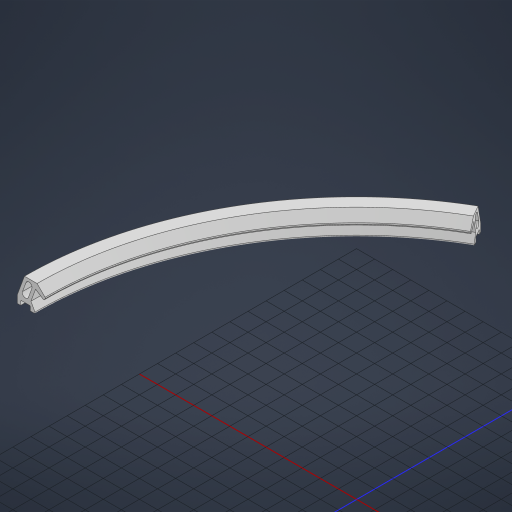
# Autodesk Inventor part: LED-Ring_Element
Saved by Autodesk Inventor 2023.2 (Build 272271030, 271C)
## iProperties
Created: 2023-02-18
Part Number: LED-Ring_Element
Material: Generisch
Document SubType Name: Modeling
Designer: Stefan
Mass: 133.438 g
Surface Area: 652.824 cm^2
Volume: 133.438 cm^3
Density: 1 g/cm^3
Appearance: Vorgabe
Author: Stefan
Autodesk Inventor part; units mm, degrees
ref_plane "YZ Plane" through (0, 0, 0) normal (1, 0, 0) x (0, 1, 0)
ref_plane "XZ Plane" through (0, 0, 0) normal (0, 1, 0) x (-1, 0, 0)
ref_plane "XY Plane" through (0, 0, 0) normal (0, 0, 1) x (1, 0, 0)
sketch "Skizze1" plane through (0, 0, 0) normal (0, 0, 1) x (1, 0, 0)
  arc A0 (-370.4, 125) -> (-371.4, 124) centre (-370.4, 124) ccw
  line L0 (-361.6643, 125) -> (-370.4, 125)
  arc A1 (-360.6643, 124) -> (-361.6643, 125) centre (-361.6643, 124) ccw
  line L1 (-360.6643, 120) -> (-360.6643, 124)
  arc A2 (-346.4361, 138.3117) -> (-345.027, 138.6477) centre (-345.8915, 139.1504) ccw
  line L2 (-344.2357, 140.0086) -> (-345.027, 138.6477)
  arc A3 (-344.2357, 140.0086) -> (-344.3931, 141.2184) centre (-345.1002, 140.5113) ccw
  line L3 (-353.1746, 150) -> (-344.3931, 141.2184)
  line L4 (-367.1746, 150) -> (-353.1746, 150)
  line L5 (-375, 128.5) -> (-367.1746, 150)
  line L6 (-375, 120) -> (-375, 128.5)
  line L7 (-371.4, 120) -> (-375, 120)
  line L8 (-371.4, 124) -> (-371.4, 120)
  line L9 (-357.3008, 147) -> (-364.6666, 147) construction
  line L10 (-364.6666, 147) -> (-371.4, 128.5) construction
  line L11 (0, 0) -> (-360, 0) construction
  line L12 (-356.9218, 138.1504) -> (-345, 0) construction
  line L13 (-356.9218, 138.1504) -> (0, 138.1504) construction
  line L14 (0, 138.1504) -> (0, 0) construction
  line L15 (-360, 129.6932) -> (-360, 0) construction
  line L16 (0, 0) -> (-225, 0) construction
  line L17 (-225, 0) -> (-225, 50) construction
  line L18 (-225, 50) -> (0, 50) construction
  line L19 (0, 50) -> (0, 0) construction
  line L20 (-346.4361, 138.3117) -> (-354.8697, 143.7886)
  line L21 (-360, 129.6932) -> (-355.5655, 121.4749)
  arc A4 (-356.4455, 120) -> (-355.5655, 121.4749) centre (-356.4455, 121) ccw
  line L22 (-225, 0) -> (-345, 0) construction
  line L23 (-345, 0) -> (-345, 35) construction
  line L24 (-345, 35) -> (-225, 35) construction
  line L25 (-225, 35) -> (-225, 0) construction
  line L26 (-356.4455, 120) -> (-360.6643, 120)
  line L27 (-354.8697, 143.7886) -> (-360, 129.6932)
  line L28 (-356.9218, 138.1504) -> (0, 8.2415) construction
  line L29 (-363.6, 129.6932) -> (-357.3008, 147) construction
  line L30 (-360, 129.6932) -> (-374.5657, 129.6932) construction
  line L31 (-363.6, 129.6932) -> (-358.3696, 120) construction
  line L32 (-344.2357, 140.0086) -> (-355.581, 120.4973) construction
  arc A5 (-358.9913, 142.3556) -> (-365.4954, 144.7229) centre (-362.2433, 143.5392) ccw
  arc A6 (-369.2753, 134.3376) -> (-362.7712, 131.9703) centre (-366.0232, 133.1539) ccw
  line L33 (-365.4954, 144.7229) -> (-369.2753, 134.3376)
  line L34 (-358.9913, 142.3556) -> (-362.7712, 131.9703)
  line L35 (-371.4, 120) -> (-371.4, 128.5) construction
  dimension "d1" = 30
  dimension "d5" = 1
  dimension "d6" = 1
  dimension "d9" = 135
  dimension "d14" = 8.5
  dimension "d18" = 360
  dimension "d25" = 50
  dimension "d26" = 225
  dimension "d31" = 14
  dimension "d40" = 3.5
  dimension "d41" = 120
  dimension "d42" = 35
  dimension "d43" = 1
  dimension "d47" = 6
  dimension "d50" = 65.068
  dimension "d54" = 15
  dimension "d55" = 3
  dimension "d59" = 12
  dimension "d60" = 160
  dimension "d61" = 120
  dimension "d63" = 3.6
  dimension "d64" = 3.6
  dimension "d65" = 5
  dimension "d66" = 15
  constraints: 72 end point, 19 tangent, 15 point on circle, 12 point on line, 8 parallel, 7 centre point, 6 horizontal, 5 vertical, 3 perpendicular, 2 collinear, 2 equal radius, 1 horizontal alignment, 4 other
  measures "d1" distance between parallel lines of L7 L4
  measures "d5" radius of A3
  measures "d6" radius of A0
  measures "d9" angle of L3 L4
  measures "d14" distance of L6.start L5.start
  measures "d18" distance of L11.end L11.start
  measures "d25" distance of L16.end L17.end
  measures "d26" distance of L17.end L18.end
  measures "d31" distance of L4.start L3.start
  measures "d40" distance from line of L20.start L3
  measures "d41" distance of L23.end L24.end
  measures "d42" distance of L22.end L23.end
  measures "d43" radius of A4
  measures "d47" distance of L20.end L13.start
  measures "d54" distance of L15.start L20.end
  measures "d55" distance between parallel lines of L4 L9
  measures "d59" angle of L3 L20
  measures "d60" angle of L15 L27
  measures "d61" distance between parallel lines of L11 L26
  measures "d63" distance of L15.start L29.start
  measures "d64" distance between parallel lines of L8 L6
  measures "d65" distance between parallel lines of L0 L7
  measures "d66" distance between parallel lines of L15 L6
revolve "Umdrehung1" add sketch "Skizze1" angle 60 about axis through (0, 138.1504, 0) along (0, -1, 0)
